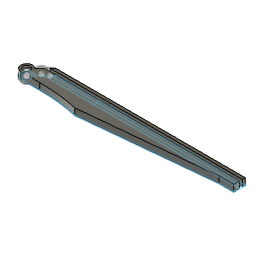
Finger1Section4P2V1 (Autodesk Fusion 360 design; units mm, degrees)
Autodesk Fusion 360 part; units mm, degrees
sketch "Sketch1" plane through (0, 0, 0) normal (0, 0, 1) x (1, 0, 0)
  circle A0 centre (0.507, 0) radius 1.25
  line L0 (3.507, 3) -> (2.507, 3)
  line L1 (4.507, 4) -> (5.507, 5)
  line L2 (5.507, 5) -> (20.507, 5)
  arc A1 (1.9212, 1.4142) -> (0.507, -2) centre (0.507, 0) ccw
  line L3 (1.9212, 1.4142) -> (3.507, 3)
  line L4 (20.507, 4) -> (4.507, 4)
  line L5 (20.507, 3) -> (3.507, 3)
  line L6 (20.507, 5) -> (70.507, 5)
  line L7 (20.507, 4) -> (70.507, 4)
  line L8 (20.507, 3) -> (70.507, 3)
  line L9 (70.507, 3) -> (70.507, 1)
  line L10 (70.507, 5) -> (70.507, 4)
  line L11 (70.507, 1) -> (65.507, 1)
  line L12 (65.507, 1) -> (20.507, -3.5)
  line L13 (7.007, -2) -> (0.507, -2)
  arc A2 (20.507, -3.5) -> (7.007, -2) centre (7.007, -63.5) ccw
  dimension "d3" = 2.5
  dimension "d7" = 4
  dimension "d14" = 1
  dimension "d15" = 1
  dimension "d17" = 50
  dimension "d18" = 50
  dimension "d19" = 50
  dimension "d20" = 2
  dimension "d24" = 5
  constraint horizontal L0
  constraint concentric A0 A1
  constraint coincident L1 L4.end
  constraint parallel L2 L4
  constraint coincident L3 L0.start
  constraint parallel L0 L5
  constraint perpendicular L9 L11
  constraint tangent L13 A2
  measures "d3" diameter of A0
  measures "d7" diameter of A1
  measures "d14" distance of L2 L4
  measures "d15" distance of L4 L5
  measures "d17" distance of L5.start L8.end
  measures "d18" distance of L4.start L7.end
  measures "d19" distance of L2.end L6.end
  measures "d20" distance of L8.end L9.end
  measures "d24" distance of L9.end L11.end
extrude "Extrude4" add sketch "Sketch1" along normal blind 2.2 contours A1 L3 L5 L8 L9 L11 L12 L13 A2 makes body 1
extrude "Extrude5" add sketch "Sketch1" along normal blind 2.2 separate body contours L1 L2 L4 L6 L7 L10 makes body 2
